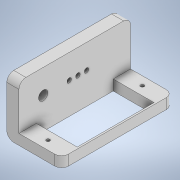
# Autodesk Inventor part: Part4
Saved by Autodesk Inventor 2021 (Build 250183000, 183)
## iProperties
Created: 2021-10-11
Part Number: Part4
Material: Generic
Document SubType Name: Modeling
Designer: Route
Density: 1 g/cm^3
Appearance: Default
Author: Route
Autodesk Inventor part; units mm, degrees
ref_plane "YZ Plane" through (0, 0, 0) normal (1, 0, 0) x (0, 1, 0)
ref_plane "XZ Plane" through (0, 0, 0) normal (0, 1, 0) x (-1, 0, 0)
ref_plane "XY Plane" through (0, 0, 0) normal (0, 0, 1) x (1, 0, 0)
sketch "Sketch1" plane through (0, 0, 0) normal (0, 1, 0) x (-1, 0, 0)
  line L0 (12.8, 0) -> (12.8, 32.2)
  line L1 (12.8, 16.1) -> (0, 16.1)
  line L2 (0, 0) -> (0, 32.2)
  line L3 (6.4, 27.2) -> (12.3, 27.2)
  line L4 (12.3, 27.2) -> (12.3, 5)
  line L5 (12.3, 5) -> (0.5, 5)
  line L6 (0.5, 5) -> (0.5, 27.2)
  line L7 (0.5, 27.2) -> (6.4, 27.2)
  line L8 (0, 0) -> (12.8, 0)
  circle A0 centre (6.4, 2.5) radius 0.5
  line L9 (0, 32.2) -> (12.8, 32.2)
  circle A1 centre (6.4, 29.7) radius 0.5
  line L10 (12.8, 32.2) -> (15.8, 32.2)
  line L11 (15.8, 32.2) -> (15.8, 0)
  line L12 (15.8, 0) -> (12.8, 0)
  line L13 (12.8, 0) -> (12.8, 32.2)
  point P0 (0, 0)
  dimension "d0" = 5.9
  dimension "d1" = 11.8
  dimension "d2" = 1
  dimension "d3" = 1
  dimension "d4" = 3
  constraints: 28 end point, 5 perpendicular, 2 centre point, 2 midpoint, 2 parallel, 1 horizontal, 1 point on line
  measures "d0" distance of L3.start L3.end
  measures "d1" distance of L4.end L5.end
  measures "d2" diameter of A0
  measures "d3" diameter of A1
  measures "d4" distance of L11.end L12.end
extrude "Extrusion1" add sketch "Sketch1" along normal blind 3 contours L8 L2 L1 L6 L5 L4 L0 | L0 L10 L11 L12 | L1 L4 L3 L7 L6 L2 L9 L0
sketch "Sketch2" plane through (0, 3, 0) normal (0, 1, 0) x (1, 0, 0)
  line L0 (-15.8, 0) -> (-15.8, -32.2) projected
  line L1 (0, 0) -> (-15.8, 0) projected
  line L2 (-15.8, -32.2) -> (-12.3, -32.2)
  line L3 (-12.3, -32.2) -> (-12.3, 0)
  line L4 (-12.3, 0) -> (-15.8, 0)
  line L5 (-15.8, 0) -> (-15.8, -32.2)
  dimension "d7" = 3.5
  constraints: 8 end point, 2 parallel, 1 horizontal, 1 perpendicular, 1 point on line
  measures "d7" distance of L4.end L3.end
extrude "Extrusion2" add sketch "Sketch2" along normal blind 13
fillet "Fillet1" radius 2 1 edges at (-15.8, 0, 16.1)
sketch "Sketch3" plane through (-15.8, 16, 0) normal (-1, 0, 0) x (0, 0, 1)
  line L0 (32.2, -14) -> (32.2, 0) projected
  line L1 (32.2, -14) -> (0, -14) projected
  line L2 (32.2, 0) -> (51.999, 0) construction
  circle A0 centre (25.2, -7) radius 1.35
  line L3 (25.2, -7) -> (32.7, -7) construction
  circle A1 centre (17.7, -7) radius 0.65
  circle A2 centre (15.2, -7) radius 0.65
  circle A3 centre (12.7, -7) radius 0.65
  point P0 (0, -16)
  dimension "d12" = 2.7
  dimension "d17" = 1.3
  dimension "d18" = 1.3
  dimension "d19" = 1.3
  constraints: 4 centre point, 4 end point, 2 horizontal
  measures "d12" diameter of A0
  measures "d17" diameter of A1
  measures "d18" diameter of A2
  measures "d19" diameter of A3
extrude "Extrusion3" cut sketch "Sketch3" against normal blind 13
fillet "Fillet2" radius 2 4 edges at (-14.05, 16, 0) (-14.05, 16, 32.2) (0, 1.5, 32.2) (0, 1.5, 0)
body "Solid1"
